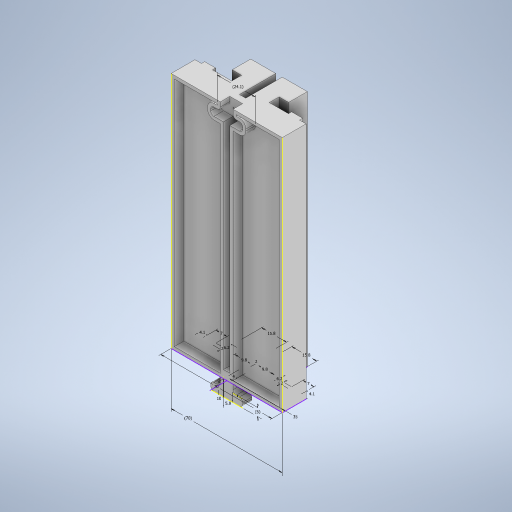
# Autodesk Inventor part: 밑판(미니)
Saved by Autodesk Inventor 2023 (Build 270158000, 158)
## iProperties
Created: 2023-04-28
Part Number: 밑판(미니)
Material: 일반
Document SubType Name: Modeling
Designer: rlatk
Density: 1 g/cm^3
Appearance: 기본값
Author: rlatk
Autodesk Inventor part; units mm, degrees
ref_plane "YZ Plane" through (0, 0, 0) normal (1, 0, 0) x (0, 1, 0)
ref_plane "XZ Plane" through (0, 0, 0) normal (0, 1, 0) x (-1, 0, 0)
ref_plane "XY Plane" through (0, 0, 0) normal (0, 0, 1) x (1, 0, 0)
sketch "스케치1" plane through (0, 0, 0) normal (0, 1, 0) x (-1, 0, 0)
  line L0 (-17.8, -18) -> (-17.8, -6.2)
  line L1 (-11.8155, 0) -> (11.8052, 0)
  line L2 (17.8, -6.2) -> (17.8, -17.9333)
  line L3 (11.8052, 0) -> (11.7948, -6.2)
  line L4 (11.7948, -6.2) -> (17.8, -6.2)
  line L5 (-11.8155, 0) -> (-11.7845, -6.2)
  line L6 (-11.7845, -6.2) -> (-17.8, -6.2)
  line L7 (-35.0051, 0) -> (-35.0051, 15)
  line L8 (-35.0051, 15) -> (34.9949, 15)
  line L9 (34.9949, 15) -> (34.9949, 0)
  line L10 (-2, -18) -> (-2, 5)
  line L11 (-2, 5) -> (2, 5)
  line L12 (2, 5) -> (2, -17.9333)
  line L13 (17.8, -17.9333) -> (2, -17.9333)
  line L14 (-2, -18) -> (-17.8, -18)
  line L15 (34.9949, 0) -> (30.8949, 0)
  line L16 (23.7949, 0) -> (-23.8051, 0)
  line L17 (-30.9051, 0) -> (-35.0051, 0)
  line L18 (-0.0051, 0) -> (-0.0051, 25.9263)
  line L19 (-30.9051, 0) -> (-23.8051, 0)
  line L20 (30.8949, 0) -> (23.7949, 0)
  line L21 (-30.9051, 0) -> (-23.9051, 0)
  line L22 (-23.9051, 0) -> (-23.9051, -2)
  line L23 (-23.9051, -2) -> (-30.9051, -2)
  line L24 (-30.9051, -2) -> (-30.9051, 0)
  line L25 (30.8949, 0) -> (23.8949, 0)
  line L26 (23.8949, 0) -> (23.8949, -2)
  line L27 (23.8949, -2) -> (30.8949, -2)
  line L28 (30.8949, -2) -> (30.8949, 0)
  point P0 (0, 0)
  point P1 (0, 0)
  point P2 (-14.7922, -6.2)
  point P3 (0, 5)
  point P4 (11.8052, 0)
  point P5 (-11.8155, 0)
  point P6 (17.8, -12.0667)
  point P7 (14.7974, -6.2)
  point P8 (11.8, -3.1)
  point P9 (-11.8, -3.1)
  point P10 (-0.0051, 15)
  point P11 (-2, 0)
  point P12 (2, 0)
  point P13 (11.8052, 0)
  point P14 (-30.9051, -1)
  point P15 (30.8949, -1)
  point P16 (23.8949, 0)
  point P17 (-23.9051, 0)
  dimension "d5" = 70
  dimension "d11" = 4
  dimension "d25" = 15.8
  dimension "d26" = 15.8
  dimension "d28" = 2
  dimension "d29" = 6.2
  dimension "d30" = 6.2
  dimension "d31" = 9.8
  dimension "d32" = 9.8
  dimension "d74" = 35
  dimension "d78" = 7
  dimension "d79" = 2
  dimension "d80" = 7
  dimension "d81" = 2
  dimension "d82" = 4.1
  dimension "d83" = 4.1
  constraints: 58 end point, 12 parallel, 11 midpoint, 8 horizontal, 7 perpendicular, 2 point on line, 1 coincident, 1 collinear, 1 vertical
  measures "d5" distance of L7.end L8.end
  measures "d11" distance of L10.end L11.end
  measures "d25" distance between parallel lines of L10 L0
  measures "d26" distance from line of point (17.8, -12.067) L12
  measures "d28" distance from line of L12 point (0, 0)
  measures "d29" distance between parallel lines of L6 L16
  measures "d30" distance from line of point (14.797, -6.2) L16
  measures "d31" distance from line of L12 point (11.8, -3.1)
  measures "d32" distance from line of L10 point (-11.8, -3.1)
  measures "d74" distance between parallel lines of L7 L18
  measures "d78" distance of L22.end L23.end
  measures "d79" distance of L21.end L22.end
  measures "d80" distance of L27.end L26.end
  measures "d81" distance of L26.end L25.end
  measures "d82" distance from line of L7 point (-30.905, -1)
  measures "d83" distance from line of L9 point (30.895, -1)
extrude "돌출1" add sketch "스케치1" along normal blind 150 contours L0 L6 L5 L1 L10 L14 | L1 L16 L19 L17 L7 L8 L18 L11 L10 | L12 L11 L18 L8 L9 L15 L20 L16 L1 | L1 L3 L4 L2 L13 L12
sketch "스케치2" plane through (-34.9949, 0, 15) normal (0, 0, 1) x (1, 0, 0)
  line L0 (32.9949, 0) -> (32.9949, 150) projected
  line L1 (36.9949, 0) -> (36.9949, 150) projected
  line L2 (32.9949, 150) -> (36.9949, 150)
  line L3 (36.9949, 150) -> (36.9949, 0)
  line L4 (36.9949, 0) -> (32.9949, 0)
  line L5 (32.9949, 0) -> (32.9949, 150)
  line L6 (32.9949, 5) -> (36.9949, 5)
  line L7 (32.9949, 145) -> (36.9949, 145)
  point P0 (34.9949, 0)
  point P1 (34.9949, 0)
  point P2 (34.9949, 5)
  point P3 (34.9949, 150)
  point P4 (34.9949, 145)
  point P5 (36.9949, 145)
  point P6 (32.9949, 145)
  dimension "d21" = 5
  dimension "d22" = 5
  constraints: 12 end point, 5 point on line, 4 midpoint, 3 perpendicular, 2 parallel, 1 horizontal
  measures "d21" distance of point (34.995, 0) point (34.995, 5)
  measures "d22" distance of point (34.995, 150) point (34.995, 145)
extrude "돌출2" cut sketch "스케치2" against normal blind 10 contours L0 L7 L1 L6
sketch "스케치4" plane through (-2, 0, 5) normal (1, 0, 0) x (0, 0, -1)
  line L0 (-10, 0) -> (-4.2, 0)
  line L1 (-4.2, 0) -> (-4.2, -10)
  line L2 (-4.2, -10) -> (-10, -10)
  line L3 (-10, -10) -> (-10, 0)
  line L4 (-4.2, -5) -> (-10, -5)
  point P0 (5, 0)
  dimension "d33" = 5.8
  dimension "d34" = 10
  constraints: 10 end point, 2 midpoint, 2 parallel, 1 horizontal, 1 perpendicular
  measures "d33" distance of L1.end L2.end
  measures "d34" distance between parallel lines of L2 L0
extrude "돌출3" add sketch "스케치4" along normal blind 6 and the other way blind 2
extrude "돌출4" add sketch "스케치4" along normal blind 12 and the other way blind 8 contours L4 L1 L2 L3
sketch "스케치5" plane through (-34.9949, 150, 15) normal (0, 0, 1) x (1, 0, 0)
  line L0 (0, 0) -> (70, 0) projected
  line L1 (39, 0) -> (31, 0)
  line L2 (31, 0) -> (31, -9.9)
  line L3 (31, -9.9) -> (39, -9.9)
  line L4 (39, -9.9) -> (39, 0)
  line L5 (39, -4.95) -> (31, -4.95)
  line L6 (45.05, -4.8) -> (24.95, -4.8)
  line L7 (24.95, -4.8) -> (24.95, -9.9)
  line L8 (24.95, -9.9) -> (45.05, -9.9)
  line L9 (45.05, -9.9) -> (45.05, -4.8)
  point P0 (34.9949, -150)
  point P1 (35, 0)
  point P2 (35, -9.9)
  point P3 (39, -4.8)
  point P4 (31, 0)
  point P5 (31, -4.8)
  dimension "d43" = 8
  dimension "d44" = 9.9
  dimension "d45" = 20.1
  dimension "d48" = 5.1
  constraints: 18 end point, 6 midpoint, 4 parallel, 2 horizontal, 2 perpendicular, 1 point on line
  measures "d43" distance of L3.end L2.end
  measures "d44" distance of L2.end L1.end
  measures "d45" distance of L8.end L7.end
  measures "d48" distance between parallel lines of L6 L8
extrude "돌출5" cut sketch "스케치5" against normal blind 6
sketch "스케치6" plane through (-34.9949, 0, 15) normal (0, 0, 1) x (1, 0, 0)
  line L0 (38.9949, -5) -> (44.9949, -5) projected
  line L1 (24.9949, -10) -> (44.9949, -10) projected
  point P0 (34.9949, 0)
  point P1 (41.9949, -5)
  dimension "d49" = 5
  constraints: 1 midpoint
  measures "d49" distance from line of point (41.995, -5) L1
fillet "모깎기1" radius 2 4 edges at (10, -10, 12.1) (10, -5, 12.1) (-10, -10, 12.1) (-10, -5, 12.1)
fillet "모깎기2" radius 2 8 edges at (-10.0449, 145.2, 12) (10.0551, 145.2, 12) (-10.0449, 140.1, 12) (10.0551, 140.1, 12) (-3.9949, 145.2, 12) (4.0051, 145.2, 12) (-4, -5, 12.1) (4, -5, 12.1)
sketch "스케치8" plane through (4, 0, 9.2) normal (0, 0, -1) x (-1, 0, 0)
  point P0 (4, 0)
sketch "스케치9" plane through (-34.9949, 0, 15) normal (0, 0, 1) x (1, 0, 0)
  line L0 (0, 0) -> (0, 150) projected
  line L1 (70, 0) -> (70, 150) projected
  point P0 (34.9949, 0)
  dimension "d58" = 70
  measures "d58" distance between parallel lines of L0 L1
sketch "스케치15" plane through (-34.9949, 0, 15) normal (0, 0, 1) x (1, 0, 0)
  arc A0 (39, 147.2) -> (41, 145.2) centre (41, 147.2) ccw projected
  line L0 (41, 145.2) -> (43.05, 145.2) projected
  arc A1 (45.05, 143.2) -> (43.05, 145.2) centre (43.05, 143.2) ccw projected
  line L1 (45.05, 143.2) -> (45.05, 142.1) projected
  arc A2 (43.05, 140.1) -> (45.05, 142.1) centre (43.05, 142.1) ccw projected
  line L2 (43.05, 140.1) -> (36.9949, 140.1) projected
  line L3 (36.9949, 140.1) -> (36.9949, 5) projected
  line L4 (36.9949, 5) -> (32.9949, 5) projected
  line L5 (32.9949, 5) -> (32.9949, 140.1) projected
  line L6 (32.9949, 140.1) -> (26.95, 140.1) projected
  arc A3 (24.95, 142.1) -> (26.95, 140.1) centre (26.95, 142.1) ccw projected
  line L7 (24.95, 142.1) -> (24.95, 143.2) projected
  arc A4 (26.95, 145.2) -> (24.95, 143.2) centre (26.95, 143.2) ccw projected
  line L8 (26.95, 145.2) -> (29, 145.2) projected
  arc A5 (29, 145.2) -> (31, 147.2) centre (29, 147.2) ccw projected
  line L9 (31, 147.2) -> (31, 150) projected
  line L10 (0, 150) -> (31, 150) projected
  line L11 (0, 0) -> (0, 150) projected
  line L12 (0, 0) -> (30.9949, 0) projected
  line L13 (30.9949, -3) -> (30.9949, 0) projected
  arc A6 (28.9949, -5) -> (30.9949, -3) centre (28.9949, -3) ccw projected
  line L14 (26.9949, -5) -> (28.9949, -5) projected
  arc A7 (26.9949, -5) -> (24.9949, -7) centre (26.9949, -7) ccw projected
  line L15 (24.9949, -8) -> (24.9949, -7) projected
  arc A8 (24.9949, -8) -> (26.9949, -10) centre (26.9949, -8) ccw projected
  line L16 (26.9949, -10) -> (42.9949, -10) projected
  arc A9 (42.9949, -10) -> (44.9949, -8) centre (42.9949, -8) ccw projected
  line L17 (44.9949, -7) -> (44.9949, -8) projected
  arc A10 (44.9949, -7) -> (42.9949, -5) centre (42.9949, -7) ccw projected
  line L18 (40.9949, -5) -> (42.9949, -5) projected
  arc A11 (38.9949, -3) -> (40.9949, -5) centre (40.9949, -3) ccw projected
  line L19 (38.9949, 0) -> (38.9949, -3) projected
  line L20 (38.9949, 0) -> (70, 0) projected
  line L21 (70, 0) -> (70, 150) projected
  line L22 (39, 150) -> (70, 150) projected
  line L23 (39, 150) -> (39, 147.2) projected
  line L24 (2, 148) -> (29, 148)
  line L25 (29, 148) -> (29, 147.2)
  line L26 (29, 147.2) -> (26.95, 147.2)
  arc A12 (26.95, 147.2) -> (22.95, 143.2) centre (26.95, 143.2) ccw
  line L27 (22.95, 143.2) -> (22.95, 142.1)
  arc A13 (22.95, 142.1) -> (26.95, 138.1) centre (26.95, 142.1) ccw
  line L28 (26.95, 138.1) -> (30.9949, 138.1)
  line L29 (30.9949, 138.1) -> (30.9949, 2)
  line L30 (38.9949, 2) -> (38.9949, 138.1)
  line L31 (38.9949, 138.1) -> (43.05, 138.1)
  arc A14 (43.05, 138.1) -> (47.05, 142.1) centre (43.05, 142.1) ccw
  line L32 (47.05, 142.1) -> (47.05, 143.2)
  arc A15 (47.05, 143.2) -> (43.05, 147.2) centre (43.05, 143.2) ccw
  line L33 (43.05, 147.2) -> (41, 147.2)
  line L34 (41, 147.2) -> (41, 148)
  line L35 (41, 148) -> (68, 148)
  line L36 (68, 148) -> (68, 2)
  line L37 (68, 2) -> (36.9949, 2)
  line L38 (36.9949, 2) -> (36.9949, -3)
  arc A16 (36.9949, -3) -> (40.9949, -7) centre (40.9949, -3) ccw
  line L39 (40.9949, -7) -> (42.9949, -7)
  line L40 (42.9949, -7) -> (42.9949, -8)
  line L41 (42.9949, -8) -> (26.9949, -8)
  line L42 (26.9949, -8) -> (26.9949, -7)
  line L43 (26.9949, -7) -> (28.9949, -7)
  arc A17 (28.9949, -7) -> (32.9949, -3) centre (28.9949, -3) ccw
  line L44 (32.9949, -3) -> (32.9949, 2)
  line L45 (32.9949, 2) -> (2, 2)
  line L46 (2, 2) -> (2, 148)
  line L47 (32.9949, 2) -> (36.9949, 2)
  line L48 (30.9949, 2) -> (38.9949, 2)
  point P0 (34.9949, 0)
  point P1 (34.9949, 2)
  dimension "d69" = 2
  dimension "d193" = 2
  dimension "d194" = 2
  constraints: 50 end point, 12 point on circle, 6 centre point, 2 midpoint, 1 horizontal, 1 perpendicular, 25 other
  measures "d69" distance between parallel lines of L11 L46
  measures "d193" distance between parallel lines of L30 L3
  measures "d194" distance between parallel lines of L5 L29
extrude "돌출11" cut sketch "스케치15" against normal blind 6 contours L24 L25 L26 A12 L27 A13 L28 L29 L45 L46 | L30 L31 A14 L32 A15 L33 L34 L35 L36 L37
sketch "스케치16" plane through (-34.9949, 0, 9) normal (0, 0, 1) x (1, 0, 0)
  line L0 (47.05, 142.1) -> (47.05, 143.2) projected
  line L1 (22.95, 143.2) -> (22.95, 142.1) projected
  point P0 (34.9949, 0)
  point P1 (47.05, 142.65)
  point P2 (22.95, 142.65)
  dimension "d73" = 24.1
  constraints: 2 midpoint
  measures "d73" distance of point (47.05, 142.65) point (22.95, 142.65)
extrude "돌출12" add sketch "스케치1" along normal blind 150 contours L22 L23 L24 L19 | L20 L28 L27 L26
